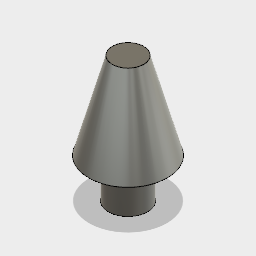
union_brazo-soporte (Autodesk Fusion 360 design; units mm, degrees)
Autodesk Fusion 360 part; units mm, degrees
sketch "Sketch1" plane through (0, 0, 0) normal (0, 0, 1) x (1, 0, 0)
  line L0 (0, 0) -> (2.5, 0)
  line L1 (2.5, 0) -> (2.5, 5)
  line L2 (2.5, 5) -> (5, 5)
  line L3 (0, 0) -> (0, 16)
  line L4 (0, 16) -> (2, 16)
  line L5 (2, 16) -> (5, 5)
revolve "Revolve1" add sketch "Sketch1" angle 360 about axis through (0, 0, 0) along (0, 1, 0)
